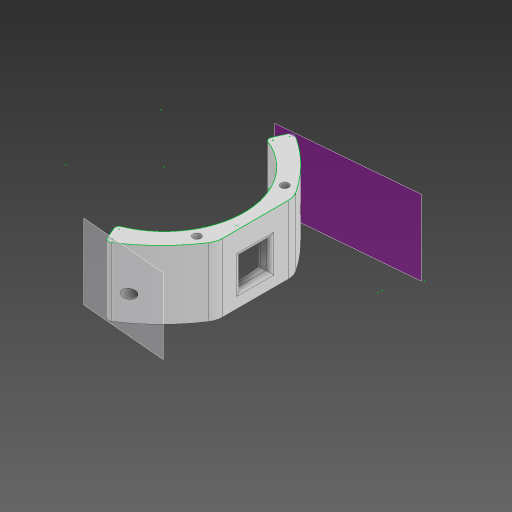
# Autodesk Inventor part: Деталь1
Saved by Autodesk Inventor 2023 (Build 270158000, 158)
## iProperties
Created: 2025-08-04
Part Number: Деталь1
Material: Типовые
Document SubType Name: Modeling
Designer: daa
Density: 1 g/cm^3
Appearance: По умолчанию
Author: daa
Autodesk Inventor part; units mm, degrees
ref_plane "YZ Plane" through (0, 0, 0) normal (1, 0, 0) x (0, 1, 0)
ref_plane "XZ Plane" through (0, 0, 0) normal (0, 1, 0) x (-1, 0, 0)
ref_plane "XY Plane" through (0, 0, 0) normal (0, 0, 1) x (1, 0, 0)
sketch "Эскиз1" plane through (0, 0, 0) normal (0, 1, 0) x (-1, 0, 0)
  arc A0 (103.6457, 54.2174) -> (103.6457, -22.3343) centre (117.1711, 15.9415) ccw
  arc A1 (103.6457, 54.2174) -> (99.1875, 64.2174) centre (6.5605, 16.9286) ccw
  arc A2 (99.1875, -32.3343) -> (103.6457, -22.3343) centre (6.5605, 14.9544) ccw
  line L0 (70.6457, 35.6756) -> (70.6457, -3.7925)
  arc A3 (99.1875, 64.2174) -> (70.6457, 35.6756) centre (143.3019, -8.4388) ccw
  arc A4 (70.6457, -3.7925) -> (99.1875, -32.3343) centre (143.3019, 40.3219) ccw
  circle A5 centre (78.0758, -6.5585) radius 2
  circle A6 centre (78.0758, 38.4415) radius 2
  point P0 (76.5758, 15.9415)
  dimension "d19" = 40.5953
  dimension "d21" = 85
  dimension "d22" = 85
  dimension "d23" = 10
  dimension "d24" = 10
  dimension "d25" = 39.4681
  dimension "d26" = 18.5418
  dimension "d27" = 33
  dimension "d28" = 33
  dimension "d29" = 18.5418
  dimension "d30" = 28.5418
  dimension "d31" = 28.5418
  dimension "d102" = 4
  dimension "d103" = 4
  dimension "d104" = 45
  dimension "d105" = 22.5
  dimension "d106" = 1.5
  constraints: 11 point on circle, 7 centre point, 2 end point, 1 vertical
  measures "d19" radius of A0
  measures "d21" radius of A3
  measures "d22" radius of A4
  measures "d23" vertical distance of A0.start A1.end
  measures "d24" vertical distance of A2.start A0.end
  measures "d25" distance of L0.start L0.end
  measures "d26" vertical distance of L0.end A0.end
  measures "d27" horizontal distance of L0.end A0.end
  measures "d28" horizontal distance of L0.start A0.start
  measures "d29" vertical distance of L0.start A0.start
  measures "d30" horizontal distance of L0.start A1.end
  measures "d31" horizontal distance of L0.end A2.start
  measures "d102" diameter of A5
  measures "d103" diameter of A6
  measures "d104" distance of A6.centre A5.centre
  measures "d105" vertical distance of point (76.576, 15.942) A5.centre
  measures "d106" horizontal distance of point (76.576, 15.942) A5.centre
extrude "Выдавливание1" add sketch "Эскиз1" along normal blind 35
sketch "Эскиз2" plane through (-70.6457, 0, 35.6756) normal (1, 0, 0) x (0, 0, -1)
  line L0 (12.234, 22.5) -> (27.234, 22.5)
  line L1 (27.234, 22.5) -> (27.234, 7.5)
  line L2 (27.234, 7.5) -> (12.234, 7.5)
  line L3 (12.234, 7.5) -> (12.234, 22.5)
  line L4 (0, 35) -> (39.4681, 35) projected
  line L5 (0, 0) -> (0, 35) projected
  point P0 (35.6756, 0)
  point P1 (0, 17.5)
  dimension "d40" = 15
  dimension "d41" = 15
  dimension "d42" = 12.5
  dimension "d44" = 12.234
  constraints: 8 end point, 2 parallel, 1 horizontal, 1 midpoint, 1 perpendicular
  measures "d40" distance of L1.end L2.end
  measures "d41" distance of L0.end L1.end
  measures "d42" distance between parallel lines of L4 L0
  measures "d44" distance between parallel lines of L3 L5
extrude "Выдавливание2" cut sketch "Эскиз2" against normal blind 35
fillet "Сопряжение1" radius 2 8 edges at (-70.6457, 7.5, 15.9416) (-70.6457, 15, 23.4416) (-70.6457, 22.5, 15.9416) (-70.6457, 15, 8.4416) (-76.5758, 22.5, 15.9416) (-77.2747, 15, 8.4416) (-76.5758, 7.5, 15.9416) (-77.2747, 15, 23.4416)
ref_plane "РабПлоскость2" through (-99.3702, 0, -32.4158) normal (0.9133448, 0, 0.407187) x (0, 1, 0)
ref_plane "РабПлоскость1" through (-99.1875, 0, -32.3343) normal (0.9133448, 0, 0.407187) x (0, 1, 0)
sketch "Эскиз4" plane through (-99.3702, 0, -32.4158) normal (0.9133448, 0, 0.407187) x (0, 1, 0)
  circle A0 centre (27.5, 5.4745) radius 2
  circle A1 centre (7.5, 5.4745) radius 2
  line L0 (35, 0) -> (35, 10.9488) projected
  line L1 (0, 0) -> (0, 10.9488) projected
  line L2 (0, 0) -> (35, 0) projected
  point P0 (0, -10.8555)
  dimension "d54" = 4
  dimension "d55" = 4
  dimension "d56" = 20
  dimension "d57" = 7.5
  dimension "d58" = 7.5
  dimension "d59" = 5.4745
  constraints: 2 centre point
  measures "d54" diameter of A0
  measures "d55" diameter of A1
  measures "d56" distance of A1.centre A0.centre
  measures "d57" distance from line of L0 A0.centre
  measures "d58" distance from line of L1 A1.centre
  measures "d59" distance from line of A0.centre L2
extrude "Выдавливание4" add sketch "Эскиз4" along normal blind 5
ref_plane "РабПлоскость4" through (-103.8284, 0, 54.2988) normal (0.9133448, 0, -0.407187) x (0, 1, 0)
ref_plane "РабПлоскость3" through (-103.6457, 0, 54.2174) normal (0.9133448, 0, -0.407187) x (0, 1, 0)
sketch "Эскиз5" plane through (-103.8284, 0, 54.2988) normal (0.9133448, 0, -0.407187) x (0, 1, 0)
  circle A0 centre (27.5, 5.4743) radius 2
  circle A1 centre (7.5, 5.4743) radius 2
  line L0 (35, 0) -> (35, 10.9488) projected
  line L1 (0, 0) -> (0, 10.9488) projected
  line L2 (0, 10.9488) -> (35, 10.9488) projected
  point P0 (0, -7.3159)
  point P1 (35, 5.4744)
  dimension "d63" = 4
  dimension "d64" = 4
  dimension "d65" = 20
  dimension "d66" = 7.5
  dimension "d67" = 7.5
  dimension "d68" = 5.4745
  constraints: 2 centre point, 1 midpoint
  measures "d63" diameter of A0
  measures "d64" diameter of A1
  measures "d65" distance of A0.centre A1.centre
  measures "d66" distance of point (35, 5.474) A0.centre
  measures "d67" distance from line of L1 A1.centre
  measures "d68" distance from line of L2 A0.centre
extrude "Выдавливание5" add sketch "Эскиз5" along normal blind 5
fillet "Сопряжение2" radius 2 4 edges at (-99.1875, 17.5, -32.3343) (-103.6457, 17.5, -22.3343) (-99.1875, 17.5, 64.2174) (-103.6457, 17.5, 54.2174)
fillet "Сопряжение3" radius 10 2 edges at (-70.6457, 17.5, 35.6756) (-70.6457, 17.5, -3.7925)
ref_plane "РабПлоскость8" through (-100.1786, 0, -30.3408) normal (-0.0871557, 0, -0.9961947) x (0, 1, 0)
sketch "Эскиз10" plane through (-100.1786, 0, -30.3408) normal (-0.0871557, 0, -0.9961947) x (0, 1, 0)
  circle A0 centre (13, 12.9425) radius 2.4
  line L0 (0, 2.9425) -> (0, 25.6939) projected
  line L1 (35, 2.9425) -> (0, 2.9425) projected
  point P0 (0, 97.153)
  dimension "d87" = 4.8
  dimension "d88" = 13
  dimension "d91" = 10
  constraints: 1 centre point
  measures "d87" diameter of A0
  measures "d88" distance from line of L0 A0.centre
  measures "d91" distance from line of L1 A0.centre
extrude "Выдавливание10" cut sketch "Эскиз10" against normal blind 41.5
ref_plane "РабПлоскость9" through (-100.1786, 0, 62.2238) normal (-0.0871557, 0, 0.9961947) x (0, -1, 0)
sketch "Эскиз11" plane through (-100.1786, 0, 62.2238) normal (-0.0871557, 0, 0.9961947) x (0, -1, 0)
  circle A0 centre (-13, 7.9425) radius 2.4
  line L0 (0, 2.9425) -> (-35, 2.9425) projected
  line L1 (0, 25.6939) -> (0, 2.9425) projected
  point P0 (0, 94.3742)
  dimension "d93" = 4.8
  dimension "d94" = 5
  dimension "d95" = 13
  constraints: 1 centre point
  measures "d93" diameter of A0
  measures "d94" distance from line of A0.centre L0
  measures "d95" distance from line of L1 A0.centre
extrude "Выдавливание11" cut sketch "Эскиз11" against normal blind 11.75
sketch "Эскиз12" plane through (-91.2422, 13, 51.2107) normal (-0.0871557, 0, 0.9961947) x (0.9961947, 0, 0.0871557)
  circle A0 centre (0, 0) radius 1.25
  point P0 (86.4317, -13)
  dimension "d98" = 2.5
  constraints: 1 centre point, 2 other
  measures "d98" diameter of A0
extrude "Выдавливание12" cut sketch "Эскиз12" against normal blind 11.75
sketch "Эскиз13" plane through (0, 35, 0) normal (0, 1, 0) x (1, 0, 0)
  arc A0 (-70.6457, 0.8995) -> (-72.2916, 6.3957) centre (-80.6457, 0.8995) ccw projected
  arc A1 (-72.2916, 6.3957) -> (-97.2957, 31.1514) centre (-143.3019, -40.3219) ccw projected
  arc A2 (-97.2957, 31.1514) -> (-100.1786, 30.3408) centre (-98.3782, 29.4697) ccw projected
  arc A3 (-100.1786, 30.3408) -> (-102.894, 24.2354) centre (-6.5605, -14.9544) ccw projected
  arc A4 (-102.894, 24.2354) -> (-101.7988, 21.6307) centre (-101.0415, 23.4817) ccw projected
  arc A5 (-101.7988, -53.5137) -> (-101.7988, 21.6307) centre (-117.1711, -15.9415) ccw projected
  arc A6 (-101.7988, -53.5137) -> (-102.894, -56.1184) centre (-101.0415, -55.3648) ccw projected
  arc A7 (-102.894, -56.1184) -> (-100.1786, -62.2238) centre (-6.5605, -16.9286) ccw projected
  arc A8 (-100.1786, -62.2238) -> (-97.2957, -63.0344) centre (-98.3782, -61.3527) ccw projected
  arc A9 (-97.2957, -63.0344) -> (-72.2916, -38.2787) centre (-143.3019, 8.4388) ccw projected
  arc A10 (-72.2916, -38.2787) -> (-70.6457, -32.7826) centre (-80.6457, -32.7826) ccw projected
  line L0 (-70.6457, -32.7826) -> (-70.6457, 0.8995) projected
  point P0 (0, 0)
  point P1 (-72.6457, -23.4416)
